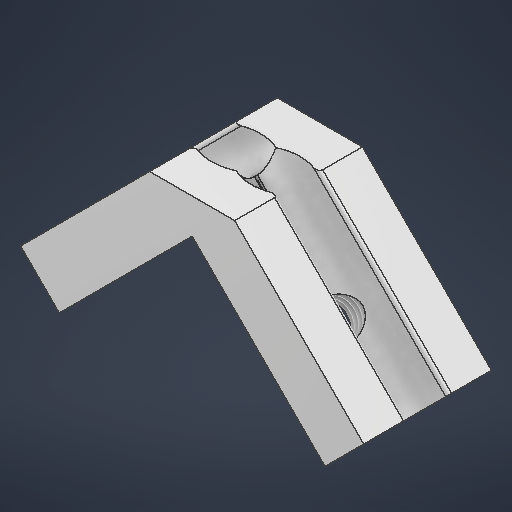
# Autodesk Inventor part: ESCUADRA UNIÓN 45 DISEÑO NUEVO V2
Saved by Autodesk Inventor 2025 (Build 290162000, 162)
## iProperties
Created: 2026-02-04
Part Number: ESCUADRA UNIÓN 45 DISEÑO NUEVO V2
Material: Aluminio
Document SubType Name: Modeling
Designer: Frank
Density: 2.7 g/cm^3
Appearance: Satinado
Author: Frank
Autodesk Inventor part; units mm, degrees
sketch "Sketch1" plane through (0, 0, 0) normal (0, 0, 1) x (1, 0, 0)
  line L0 (-7, 5.7279) -> (7, 5.7279)
  line L1 (-7, 5.7279) -> (-28.2132, -15.4853)
  line L2 (-28.2132, -15.4853) -> (-21.8492, -21.8492)
  line L3 (0, 0) -> (-21.8492, -21.8492)
  line L4 (7, 5.7279) -> (28.2132, -15.4853)
  line L5 (28.2132, -15.4853) -> (21.8492, -21.8492)
  line L6 (0, 0) -> (21.8492, -21.8492)
  line L7 (0, 15.5718) -> (0, -18.5373) construction
  dimension "d112" = 30
  dimension "d204" = 7
  dimension "d205" = 7
  dimension "d207" = 30
  dimension "d208" = 45
  dimension "d209" = 45
  dimension "d210" = 9
  dimension "d211" = 9
  constraints: 16 end point, 2 coincident, 2 perpendicular, 1 horizontal, 1 point on line, 1 vertical
  measures "d112" distance of L0.start L1.end
  measures "d204" distance from line of L7 L0.end
  measures "d205" distance from line of L7 L0.start
  measures "d207" distance from line of L5 L0.end
  measures "d208" angle of L7 L3
  measures "d209" angle of L6 L7
  measures "d210" distance between parallel lines of L3 L1
  measures "d211" distance between parallel lines of L6 L4
extrude "Extrusion1" add sketch "Sketch1" against normal blind 21
ref_plane "Plano de trabajo1" through (0, 0, 0) normal (1, 0, 0) x (0, 0, -1)
ref_plane "Plano de trabajo2" through (28.2132, -15.4853, -21) normal (0.7071, 0.7071, 0) x (-0.7071, 0.7071, 0)
sketch "Boceto2" plane through (28.2132, -15.4853, 0) normal (0.7071, -0.7071, 0) x (-0.7071, -0.7071, 0)
  line L0 (-3.8291, 10.5) -> (9.1738, 10.5) construction
  line L1 (0, 7.5) -> (0, 13.5)
  arc A0 (0, 7.5) -> (6.6379, 10.25) centre (2.6458, 10.5) ccw
  arc A1 (6.6379, 10.75) -> (0, 13.5) centre (2.6458, 10.5) ccw
  line L2 (0, 21) -> (9, 21) projected
  line L3 (9, 0) -> (0, 0) projected
  line L4 (7.1379, 10.75) -> (7.1379, 10.25)
  line L5 (7.1379, 10.25) -> (6.6379, 10.25)
  line L6 (7.1379, 10.75) -> (6.6379, 10.75)
  point P0 (0.9314, 0)
  dimension "d163" = 6
  dimension "d164" = 3
  dimension "d167" = 4
  dimension "d171" = 10.5
  dimension "d172" = 10.5
  dimension "d179" = 0.25
  dimension "d180" = 0.5
  dimension "d181" = 0.5
  constraints: 10 end point, 4 point on circle, 3 horizontal, 2 centre point, 1 vertical
  measures "d163" distance of L1.end L1.start
  measures "d164" distance from line of L1.start L0
  measures "d167" radius of A1
  measures "d171" distance between parallel lines of L2 L0
  measures "d172" distance between parallel lines of L3 L0
  measures "d179" distance between parallel lines of L0 L6
  measures "d180" distance between parallel lines of L6 L5
  measures "d181" distance of L4.end L5.end
extrude "Extrusión2" cut sketch "Boceto2" against normal up to surface surface through (0, 0, 0) normal (1, 0, 0)
mirror "Simetría1" about plane through (0, 0, 0) normal (1, 0, 0) of "Extrusión2"
fillet "Empalme1" radius 0.5 4 edges at (17.6066, -4.8787, -7.5) (17.6066, -4.8787, -13.5) (-17.6066, -4.8787, -13.5) (-17.6066, -4.8787, -7.5)
sketch "Boceto3" plane through (28.2132, -15.4853, -21) normal (0.7071, 0.7071, 0) x (-0.7071, 0.7071, 0)
  arc A0 (30, 14.4555) -> (30.7384, 14.016) centre (30.5, 14.4555) ccw projected
  line L0 (30, 14.4555) -> (0, 14.4555) projected
  line L1 (0, 14.4555) -> (0, 14.016) projected
  line L2 (0, 14.016) -> (30.7384, 14.016) projected
  line L3 (0, 14.016) -> (30.7384, 14.016) projected
  line L4 (0, 10.75) -> (0, 14.016) projected
  arc A1 (34.9497, 13.7698) -> (30.7384, 14.016) centre (32.6458, 10.5) ccw projected
  line L5 (0, 10.75) -> (33.2616, 10.75) projected
  line L6 (0, 10.75) -> (32.7616, 10.75) projected
  line L7 (0, 10.75) -> (32.7616, 10.75) projected
  line L8 (0, 10.25) -> (0, 10.75) projected
  line L9 (0, 10.25) -> (32.7616, 10.25) projected
  line L10 (0, 10.25) -> (32.7616, 10.25) projected
  line L11 (0, 10.25) -> (33.2616, 10.25) projected
  line L12 (30.7384, 6.984) -> (0, 6.984) projected
  arc A2 (30.7384, 6.984) -> (34.9497, 7.2302) centre (32.6458, 10.5) ccw projected
  line L13 (0, 6.984) -> (0, 10.25) projected
  line L14 (0, 6.984) -> (0, 6.5445) projected
  line L15 (0, 6.5445) -> (30, 6.5445) projected
  arc A3 (30.7384, 6.984) -> (30, 6.5445) centre (30.5, 6.5445) ccw projected
  line L16 (30.7384, 6.984) -> (0, 6.984) projected
  line L17 (0, 6.5445) -> (30, 6.5445) projected
  line L18 (0, 6.5445) -> (0, 0) projected
  line L19 (30, 0) -> (0, 0) projected
  line L20 (30, 6.5445) -> (30, 0) projected
  line L21 (30, 14.4555) -> (0, 14.4555) projected
  line L22 (30, 21) -> (30, 14.4555) projected
  line L23 (0, 21) -> (30, 21) projected
  line L24 (0, 21) -> (0, 14.4555) projected
  circle A4 centre (14, 10.5) radius 3
  line L25 (32.7616, 10.25) -> (33.2616, 10.25) projected
  line L26 (32.7616, 10.25) -> (32.7616, 10.75) projected
  line L27 (33.2616, 10.75) -> (32.7616, 10.75) projected
  arc A5 (33.2616, 10.25) -> (34.9497, 7.2302) centre (37.2537, 10.5) ccw projected
  line L28 (0, 10.25) -> (33.2616, 10.25) projected
  line L29 (0, 10.75) -> (33.2616, 10.75) projected
  arc A6 (34.9497, 13.7698) -> (33.2616, 10.75) centre (37.2537, 10.5) ccw projected
  point P0 (30.8995, 21)
  dimension "d183" = 6
  dimension "d184" = 10.5
  dimension "d185" = 10.5
  dimension "d186" = 14
  constraints: 1 centre point
  measures "d183" diameter of A4
  measures "d184" distance from line of L19 A4.centre
  measures "d185" distance from line of L23 A4.centre
  measures "d186" distance from line of L18 A4.centre
hole "Agujero1" at (18.3137, -5.5858, -10.5) direction (-0.7071, -0.7071, 0) diameter 6 depth 9
mirror "Simetría2" about plane through (0, 0, 0) normal (1, 0, 0) of "Agujero1"
thread "Rosca1" size "M6x1" class "6H" standard "ANSI Metric M Profile" full length
thread "Rosca2" size "M6x1" class "6H" standard "ANSI Metric M Profile" full length
ref_plane "Plano de trabajo3" through (0, 0, -10.5) normal (0, 0, 1) x (1, 0, 0)
body "Solid1"
